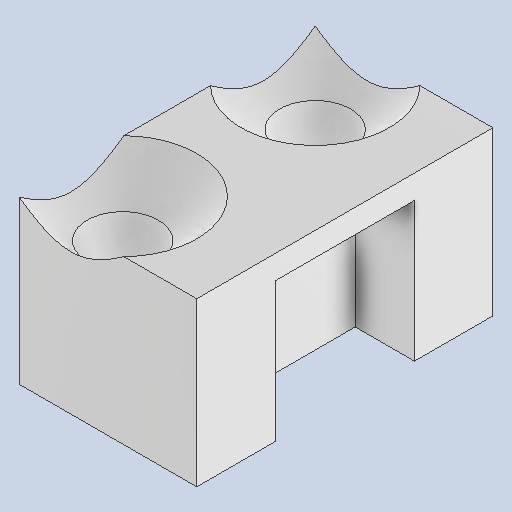
# Autodesk Inventor part: Federhalter
Saved by Autodesk Inventor 2025 (Build 290162010, 162A)
## iProperties
Created: 2024-12-03
Part Number: Federhalter
Material: PC/ABS-Kunststoff, 3DDruck, PLA
Document SubType Name: Modeling
Designer: Admin
Density: 1.1 g/cm^3
Appearance: Glatt - Weiß(2)
Author: Admin
Autodesk Inventor part; units mm, degrees
ref_plane "YZ Plane" through (0, 0, 0) normal (1, 0, 0) x (0, 1, 0)
ref_plane "XZ Plane" through (0, 0, 0) normal (0, 1, 0) x (-1, 0, 0)
ref_plane "XY Plane" through (0, 0, 0) normal (0, 0, 1) x (1, 0, 0)
sketch "Skizze1" plane through (0, 0, 0) normal (0, 0, 1) x (1, 0, 0)
  line L0 (-75.636, -5) -> (-69.636, -5)
  line L1 (-69.636, -5) -> (-69.636, 5)
  line L2 (-69.636, 5) -> (-75.636, 5)
  line L3 (-75.636, 5) -> (-75.636, -5)
  line L4 (-72.636, -5) -> (-72.636, 0) construction
  line L5 (-72.636, 0) -> (-72.636, 5) construction
  line L6 (0, 0) -> (-72.636, 0) construction
  line L7 (-65.022, 4) -> (-65.022, -4) construction
  line L8 (-65.022, 4) -> (-65.022, -4) construction
  line L9 (-65.022, 4) -> (-65.022, -4) construction
  point P0 (-63.636, 3)
  dimension "d0" = 6
  dimension "d1" = 10
  dimension "d2" = 6
  constraints: 14 end point, 2 horizontal, 2 midpoint, 2 parallel, 1 collinear, 1 perpendicular, 1 vertical, 1 other
  measures "d0" distance of L2.end L1.end
  measures "d1" distance of L1.end L0.end
  measures "d2" distance from line of L1 point (-63.636, 3)
extrude "Extrusion1" add sketch "Skizze1" along normal blind 5.5
sketch "Skizze2" plane through (-69.636, -5, 0) normal (1, 0, 0) x (0, 0, -1)
  line L0 (0, 2.65) -> (-4.7, 2.65)
  line L1 (-4.7, 2.65) -> (-4.7, 7.35)
  line L2 (-4.7, 7.35) -> (0, 7.35)
  line L3 (0, 7.35) -> (0, 2.65)
  line L4 (0, 5) -> (-4.7, 5)
  line L5 (0, 0) -> (0, 10) projected
  point P0 (0, 5)
  dimension "d5" = 4.7
  dimension "d6" = 4.7
  constraints: 10 end point, 3 midpoint, 2 horizontal, 2 parallel, 1 perpendicular
  measures "d5" distance of L1.end L2.end
  measures "d6" distance of L0.end L1.end
extrude "Extrusion2" cut sketch "Skizze2" against normal blind 2
sketch "Skizze3" plane through (0, 0, 5.5) normal (0, 0, 1) x (1, 0, 0)
  line L0 (-75.636, 5) -> (-75.636, -5) projected
  line L1 (-73.886, -3.25) -> (-75.636, -3.25) construction
  line L2 (-73.886, 3.25) -> (-75.636, 3.25) construction
  line L3 (-73.886, -3.25) -> (-73.886, -5) construction
  line L4 (-73.886, 3.25) -> (-73.886, 5) construction
  line L5 (-75.636, -5) -> (-69.636, -5) construction
  line L6 (-69.636, 5) -> (-75.636, 5) construction
  point P0 (0, 0)
  dimension "d9" = 1.75
  constraints: 8 end point, 4 point on line, 3 equal length, 2 perpendicular, 2 vertical
  measures "d9" distance from line of L0 L1.start
hole "Bohrung1" at (-73.886, 3.25, 5.5) at (-73.886, -3.25, 5.5) direction (0, 0, -1) diameter 2.4 end through all countersink diameter 5 countersink angle 90 clearance for "Flachkopfmaschinenschraube" size "M2" standard "ANSI Metrisches M Profil"
